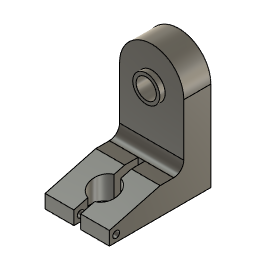
Ejercicio02jaalobuela (Autodesk Fusion 360 design; units mm, degrees)
Autodesk Fusion 360 part; units mm, degrees
sketch "Sketch1" plane through (0, 0, 0) normal (1, 0, 0) x (0, 1, 0)
  line L0 (135, 65) -> (135, -67.5)
  line L1 (135, -67.5) -> (40, -67.5)
  line L2 (40, -67.5) -> (40, 65)
  arc A0 (135, 65) -> (40, 65) centre (87.5, 65) ccw
  dimension "d1" = 95
  dimension "d2" = 132.5
  constraint vertical L0
  constraint horizontal L1
  constraint vertical L2
  measures "d1" distance of L2.end L0.start
  measures "d2" distance of L2.end L1.end
extrude "Extrude1" add sketch "Sketch1" along normal blind 40 makes body 1
sketch "Sketch2" plane through (0, 0, 0) normal (1, 0, 0) x (0, 1, 0)
  circle A0 centre (185, 85) radius 15
  circle A1 centre (185, 85) radius 20
  dimension "d5" = 30
  dimension "d6" = 40
  constraint concentric A0 A1
  measures "d5" diameter of A0
  measures "d6" diameter of A1
extrude "Extrude2" add sketch "Sketch2" along normal blind 8 separate body makes body 2
extrude "Extrude3" add sketch "Sketch2" against normal blind 40 separate body contours A0 makes body 3
hole "Hole1" at (40, 87.5, 59.3303) direction (-1, 0, 0) diameter 30 depth 60 tip angle 118 bodies 1
move_body "Move1" bodies 2 to x (1, 0, 0) y (0, 1, 0) z (0, 0, 1) at (40, -97.5, -25.6697)
box "BoxPrimitive2" add length 95 width 35 height 40 placed x (0, 1, 0) y (-1, 0, 0) z (0, 0, 1) at (270, 15, 0) separate body makes body 4
move_body "Move3" bodies 4 to x (1, 0, 0) y (0, 1, 0) z (0, 0, 1) at (-195, 25, -67.5)
sketch "Sketch5" plane through (0, 0, 0) normal (0, 1, 0) x (1, 0, 0)
  line L0 (111.4593, 23.5811) -> (111.4593, 63.5811)
  line L1 (111.4593, 63.5811) -> (186.4593, 63.5811)
  line L2 (186.4593, 63.5811) -> (186.4593, 43.5811)
  line L3 (111.4593, 23.5811) -> (186.4593, 43.5811)
  dimension "d25" = 40
  dimension "d26" = 75
  dimension "d27" = 20
  constraint vertical L0
  constraint perpendicular L0 L1
  constraint perpendicular L1 L2
  measures "d25" distance of L0.start L0.end
  measures "d26" distance of L0.end L1.end
  measures "d27" distance of L1.end L2.end
extrude "Extrude4" add sketch "Sketch5" along normal blind 95 separate body makes body 5
move_body "Move4" bodies 5 to x (1, 0, 0) y (0, 1, 0) z (0, 0, 1) at (-36.4593, 40, -3.9189)
hole "Hole2" at (140, 40, -57.5) direction (0, 1, 0) diameter 10 end through all bodies 5
sketch "Sketch6" plane through (0, 0, 0) normal (0, 0, 1) x (1, 0, 0)
  line L0 (116.4884, 241.6357) -> (116.4884, 251.6357)
  line L1 (116.4884, 241.6357) -> (95.8533, 241.6357)
  line L2 (116.4884, 251.6357) -> (95.8533, 251.6357)
  line L3 (21.4884, 246.6357) -> (21.4884, 251.6357)
  line L4 (21.4884, 246.6357) -> (21.4884, 241.6357)
  line L5 (21.4884, 241.6357) -> (57.1235, 241.6357)
  line L6 (21.4884, 251.6357) -> (57.1235, 251.6357)
  arc A0 (95.8533, 251.6357) -> (57.1235, 251.6357) centre (76.4884, 246.6357) ccw
  arc A1 (57.1235, 241.6357) -> (95.8533, 241.6357) centre (76.4884, 246.6357) ccw
  dimension "d35" = 10
  dimension "d37" = 40
  dimension "d38" = 55
  dimension "d39" = 5
  dimension "d40" = 5
  constraint vertical L0
  constraint perpendicular L0 L1
  constraint perpendicular L0 L2
  constraint perpendicular L4 L5
  constraint perpendicular L3 L6
  constraint coincident L5.end A0
  constraint concentric A0 A1
  measures "d35" distance of L0.start L0.end
  measures "d37" diameter of A0
  measures "d38" distance of A0.centre L3.start
  measures "d39" distance of L3.start L3.end
  measures "d40" distance of L3.start L4.end
extrude "Extrude5" add sketch "Sketch6" along normal blind 70 separate body makes body 6
copy_body "CopyPasteBodies1" bodies 2 5 1 4 makes body 7 makes body 8 makes body 9 makes body 10
move_body "Move5" bodies 7 8 9 10 to x (1, 0, 0) y (0, 1, 0) z (0, 0, 1) at (0, -350, 0)
combine "Combine1" operation add target body 2 tool bodies 1 5 4
copy_body "CopyPasteBodies2" bodies 6 makes body 11
move_body "Move6" bodies 11 to x (1, 0, 0) y (0, 1, 0) z (0, 0, 1) at (33.5116, -159.1357, -67.5)
combine "Combine2" operation cut target body 2 tool bodies 11
fillet "Fillet1" radius 15 1 edges at (40, 87.5, -27.5) on bodies 2
move_body "Move7" bodies 2 to x (0, -1, 0) y (1, 0, 0) z (0, 0, 1) at (-54.5, 150.5, 0)
hidden bodies 3 6 7 8 9 10
